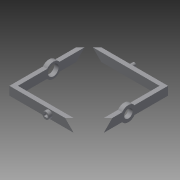
# Autodesk Inventor part: joystick_outer
Saved by Autodesk Inventor 2015 (Build 190159000, 159)
## iProperties
Created: 2015-12-08
Part Number: joystick_outer
Material: Generic
Document SubType Name: Modeling
Designer: boztalay
Density: 1 g/cm^3
Appearance: Default
Author: boztalay
Autodesk Inventor part; units mm, degrees
ref_plane "YZ Plane" through (0, 0, 0) normal (1, 0, 0) x (0, 1, 0)
ref_plane "XZ Plane" through (0, 0, 0) normal (0, 1, 0) x (-1, 0, 0)
ref_plane "XY Plane" through (0, 0, 0) normal (0, 0, 1) x (1, 0, 0)
sketch "Sketch1" plane through (0, 0, 0) normal (0, 1, 0) x (-1, 0, 0)
  line L0 (-52.705, 52.705) -> (52.705, 52.705)
  line L1 (52.705, 52.705) -> (52.705, -52.705)
  line L2 (52.705, -52.705) -> (-52.705, -52.705)
  line L3 (-52.705, -52.705) -> (-52.705, 52.705)
  line L4 (-52.705, 52.705) -> (52.705, -52.705) construction
  line L5 (52.705, 52.705) -> (-52.705, -52.705) construction
  line L6 (-59.055, 59.055) -> (59.055, 59.055)
  line L7 (59.055, 59.055) -> (59.055, -59.055)
  line L8 (59.055, -59.055) -> (-59.055, -59.055)
  line L9 (-59.055, -59.055) -> (-59.055, 59.055)
  line L10 (-59.055, 59.055) -> (59.055, -59.055) construction
  line L11 (59.055, 59.055) -> (-59.055, -59.055) construction
  point P0 (0, 0)
  dimension "d0" = 105.41
  dimension "d1" = 105.41
  dimension "d2" = 118.11
  dimension "d3" = 118.11
  constraints: 24 end point, 4 midpoint, 4 parallel, 2 horizontal, 2 perpendicular
  measures "d0" distance of L0.end L1.end
  measures "d1" distance of L1.end L2.end
  measures "d2" distance of L6.end L7.end
  measures "d3" distance of L7.end L8.end
extrude "Extrusion1" add sketch "Sketch1" along normal blind 12.7
sketch "Sketch2" plane through (-59.055, 0, -59.055) normal (-1, 0, 0) x (0, 0, 1)
  circle A0 centre (59.055, 6.35) radius 11.1125
  line L0 (0, 0) -> (0, 12.7) construction
  line L1 (0, 6.35) -> (59.055, 6.35) construction
  line L2 (59.055, 6.35) -> (118.11, 6.35) construction
  line L3 (118.11, 0) -> (118.11, 12.7) construction
  point P0 (59.055, 0)
  dimension "d6" = 22.225
  constraints: 4 end point, 2 midpoint, 1 centre point, 1 collinear, 1 horizontal
  measures "d6" diameter of A0
extrude "Extrusion2" add sketch "Sketch2" against normal up to surface (6.35 mm away)
sketch "Sketch3" plane through (-59.055, 0, -59.055) normal (-1, 0, 0) x (0, 0, 1)
  circle A0 centre (59.055, 6.35) radius 7.9375
  line L0 (0, 0) -> (0, 12.7) construction
  line L1 (0, 6.35) -> (59.055, 6.35) construction
  line L2 (59.055, 6.35) -> (118.11, 6.35) construction
  line L3 (118.11, 0) -> (118.11, 12.7) construction
  point P0 (59.055, 0)
  dimension "d9" = 15.875
  constraints: 4 end point, 2 midpoint, 1 centre point, 1 collinear, 1 horizontal
  measures "d9" diameter of A0
extrude "Extrusion3" cut sketch "Sketch3" against normal up to next
sketch "Sketch4" plane through (59.055, 0, 59.055) normal (1, 0, 0) x (0, 0, -1)
  circle A0 centre (59.055, 6.35) radius 11.1125
  line L0 (0, 0) -> (0, 12.7) construction
  line L1 (0, 6.35) -> (59.055, 6.35) construction
  line L2 (59.055, 6.35) -> (118.11, 6.35) construction
  line L3 (118.11, 0) -> (118.11, 12.7) construction
  point P0 (59.055, 0)
  dimension "d24" = 22.225
  constraints: 4 end point, 4 midpoint, 2 point on line, 1 centre point, 1 collinear, 1 horizontal
  measures "d24" diameter of A0
extrude "Extrusion4" add sketch "Sketch4" against normal up to surface (6.35 mm away)
sketch "Sketch5" plane through (59.055, 0, 59.055) normal (1, 0, 0) x (0, 0, -1)
  circle A0 centre (59.055, 6.35) radius 6.35
  line L0 (0, 0) -> (0, 12.7) construction
  line L1 (0, 6.35) -> (59.055, 6.35) construction
  line L2 (59.055, 6.35) -> (118.11, 6.35) construction
  line L3 (118.11, 0) -> (118.11, 12.7) construction
  point P0 (59.055, 0)
  dimension "d14" = 12.7
  constraints: 4 end point, 2 midpoint, 1 centre point, 1 collinear, 1 horizontal
  measures "d14" diameter of A0
extrude "Extrusion5" cut sketch "Sketch5" against normal up to next
sketch "Sketch6" plane through (59.055, 0, -59.055) normal (0, 0, -1) x (-1, 0, 0)
  circle A0 centre (59.055, 6.35) radius 2.794
  line L0 (0, 0) -> (0, 12.7) construction
  line L1 (0, 6.35) -> (59.055, 6.35) construction
  line L2 (59.055, 6.35) -> (118.11, 6.35) construction
  line L3 (118.11, 14.2875) -> (118.11, -1.5875) construction
  point P0 (59.055, 0)
  dimension "d17" = 5.588
  constraints: 4 end point, 2 midpoint, 1 centre point, 1 collinear, 1 horizontal
  measures "d17" diameter of A0
extrude "Extrusion6" add sketch "Sketch6" along normal blind 10.795
sketch "Sketch7" plane through (-59.055, 0, 59.055) normal (0, 0, 1) x (1, 0, 0)
  arc A0 (61.5154, 4.3432) -> (56.5946, 4.3432) centre (59.055, 6.35) ccw
  circle A1 centre (59.055, 6.35) radius 5.08
  line L0 (56.5946, 4.3432) -> (61.5154, 4.3432)
  line L1 (118.11, 0) -> (118.11, 12.7) construction
  line L2 (118.11, 6.35) -> (59.055, 6.35) construction
  line L3 (59.055, 6.35) -> (0, 6.35) construction
  line L4 (0, 0) -> (0, 12.7) construction
  point P0 (59.055, 0)
  dimension "d20" = 6.35
  dimension "d21" = 10.16
  constraints: 6 end point, 2 centre point, 2 midpoint, 2 point on circle, 1 coincident, 1 collinear, 1 horizontal
  measures "d20" diameter of A0
  measures "d21" diameter of A1
extrude "Extrusion7" add sketch "Sketch7" along normal blind 6.985
body "Solid1"
